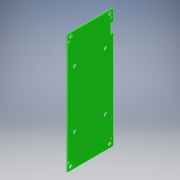
# Autodesk Inventor part: SP01
Saved by Autodesk Inventor 2022 (Build 260153000, 153)
## iProperties
Created: 2021-09-09
Part Number: SP01
Material: Acetal Resin, Black
Document SubType Name: Modeling
Designer: Bowen O'Steen
Density: 1.425 g/cm^3
Appearance: Dark Green
Author: Bowen O'Steen
Autodesk Inventor part; units mm, degrees
ref_plane "YZ Plane" through (0, 0, 0) normal (1, 0, 0) x (0, 1, 0)
ref_plane "XZ Plane" through (0, 0, 0) normal (0, 1, 0) x (-1, 0, 0)
ref_plane "XY Plane" through (0, 0, 0) normal (0, 0, 1) x (1, 0, 0)
sketch "Sketch1" plane through (0, 0, 0) normal (1, 0, 0) x (0, 1, 0)
  line L0 (50, 41.5) -> (-50, 41.5)
  line L1 (-50, 41.5) -> (-50, -41.5)
  line L2 (-50, -41.5) -> (50, -41.5)
  line L3 (50, -41.5) -> (50, 41.5)
  point P0 (0, 0)
  point P1 (50, 0)
  point P2 (0, -41.5)
  dimension "d0" = 100
  dimension "d1" = 83
  constraints: 8 end point, 2 midpoint, 2 parallel, 1 horizontal, 1 horizontal alignment, 1 perpendicular, 1 vertical alignment
  measures "d0" distance of L1.end L2.end
  measures "d1" distance of L2.end L0.start
extrude "Extrusion1" add sketch "Sketch1" along normal blind 1.6
sketch "Sketch12" plane through (0, 50, 41.5) normal (0, 1, 0) x (1, 0, 0)
  line L0 (0, 83) -> (0, 0) projected
  line L1 (0, 0) -> (1.6, 0) projected
  line L2 (1.6, 83) -> (1.6, 0) projected
  line L3 (0, 83) -> (1.6, 83) projected
  point P0 (0, 41.5)
extrude "Extrusion3" add sketch "Sketch12" along normal blind 56.75
sketch "Sketch13" plane through (0, -50, -41.5) normal (0, -1, 0) x (1, 0, 0)
  line L0 (0, 83) -> (0, 0) projected
  line L1 (0, 0) -> (1.6, 0) projected
  line L2 (1.6, 83) -> (1.6, 0) projected
  line L3 (0, 83) -> (1.6, 83) projected
  point P0 (0, 41.5)
extrude "Extrusion4" add sketch "Sketch13" along normal blind 56.75
sketch "Sketch16" plane through (0, 0, 0) normal (-1, 0, 0) x (0, 0, 1)
  line L0 (41.5, -106.75) -> (41.5, 106.75) projected
  line L1 (-41.5, 106.75) -> (41.5, 106.75) projected
  line L2 (-41.5, 106.75) -> (-41.5, -106.75) projected
  line L3 (41.5, -106.75) -> (-41.5, -106.75) projected
  line L4 (0, 0) -> (-25, 0) construction
  point P0 (35, -100.75)
  point P1 (-35, -100.75)
  point P2 (35, 100.75)
  point P3 (-35, 100.75)
  dimension "d168" = 70
  dimension "d169" = 6
  dimension "d170" = 35
  constraints: 2 end point, 2 symmetric about line, 1 horizontal, 1 horizontal alignment
  measures "d168" distance of point (-35, -100.75) point (35, -100.75)
  measures "d169" distance from line of L3 point (35, -100.75)
  measures "d170" horizontal distance of L4.start point (-35, -100.75)
hole "Hole8" at (0, -100.75, 35) at (0, -100.75, -35) at (0, 100.75, 35) at (0, 100.75, -35) direction (1, 0, 0) diameter 6 end through all
sketch "Sketch19" plane through (0, 0, 0) normal (-1, 0, 0) x (0, 0, 1)
  circle A0 centre (-27.5, 51.25) radius 3 construction
  line L0 (-39, 76.75) -> (-39, 72) construction
  line L1 (-39, 76.75) -> (-39, 81.5) construction
  line L2 (-41.5, 106.75) -> (-41.5, -106.75) construction
  line L3 (-41.5, 106.75) -> (41.5, 106.75) projected
  point P0 (0, 0)
  dimension "d194" = 4.75
  dimension "d195" = 4.75
  dimension "d203" = 25.25
  dimension "d204" = 2.5
  constraints: 4 end point, 2 coincident, 1 parallel, 1 vertical alignment
  measures "d194" distance of L0.start L0.end
  measures "d195" distance of L0.start L1.end
  measures "d203" distance from line of L3 point (-39, 81.5)
  measures "d204" distance from line of L2 point (-39, 81.5)
hole "Hole9" at (0, 72, -39) at (0, 81.5, -39) direction (1, 0, 0) diameter 2.6 end through all clearance for "Flat Head Machine Screw" size "M2" standard "Ansi Metric M Profile"
sketch "Sketch21" plane through (0, 0, 0) normal (-1, 0, 0) x (0, 0, 1)
  line L0 (-41.5, 106.75) -> (-41.5, -106.75) projected
  line L1 (-41.5, 85.75) -> (-36.5, 85.75)
  line L2 (-36.5, 85.75) -> (-36.5, 67.75)
  line L3 (-36.5, 67.75) -> (-41.5, 67.75)
  line L4 (-41.5, 67.75) -> (-41.5, 85.75)
  line L5 (-41.5, 106.75) -> (41.5, 106.75) projected
  point P0 (0, 0)
  point P1 (-41.5, 67.75)
  dimension "d205" = 5
  dimension "d206" = 21
  dimension "d207" = 18
  constraints: 8 end point, 2 parallel, 1 horizontal, 1 perpendicular, 1 point on line
  measures "d205" distance of L2.end L3.end
  measures "d206" distance between parallel lines of L5 L1
  measures "d207" distance of L1.end L2.end
extrude "Extrusion5" cut sketch "Sketch21" against normal through all
sketch "Sketch23" plane through (0, 0, 0) normal (-1, 0, 0) x (0, 0, 1)
  circle A0 centre (-35, 100.75) radius 3 projected
  line L0 (0, 0) -> (-12.2775, 0) construction
  point P0 (38, 93.75)
  point P1 (-38, 93.75)
  point P2 (38, -93.75)
  point P3 (-38, -93.75)
  dimension "d220" = 76
  dimension "d221" = 38
  dimension "d229" = 7
  constraints: 2 end point, 2 symmetric about line, 1 horizontal, 1 horizontal alignment
  measures "d220" distance of point (-38, 93.75) point (38, 93.75)
  measures "d221" horizontal distance of L0.start point (-38, 93.75)
  measures "d229" vertical distance of point (-38, 93.75) A0.centre
hole "Hole11" at (0, 93.75, 38) at (0, 93.75, -38) at (0, -93.75, 38) at (0, -93.75, -38) direction (1, 0, 0) diameter 3.454 end through all clearance for "Flat Head Machine Screw (82)" size "#4" standard "Ansi Unified Screw Threads"
sketch "Sketch24" plane through (1.6, 0, 0) normal (1, 0, 0) x (0, 0, -1)
  circle A0 centre (-38, -93.75) radius 1.727 projected
  circle A1 centre (-38, 93.75) radius 1.727 projected
  circle A2 centre (38, 93.75) radius 1.727 projected
  circle A3 centre (38, -93.75) radius 1.727 projected
  line L0 (41.5, 67.75) -> (36.5, 67.75) projected
  line L1 (36.5, 67.75) -> (36.5, 85.75) projected
  line L2 (36.5, 85.75) -> (41.5, 85.75) projected
  line L3 (41.5, 106.75) -> (41.5, 85.75) projected
  line L4 (-41.5, 106.75) -> (41.5, 106.75) projected
  line L5 (-41.5, -106.75) -> (-41.5, 106.75) projected
  line L6 (41.5, -106.75) -> (-41.5, -106.75) projected
  line L7 (41.5, 67.75) -> (41.5, -106.75) projected
  circle A4 centre (35, 100.75) radius 3 projected
  circle A5 centre (35, -100.75) radius 3 projected
  circle A6 centre (-35, -100.75) radius 3 projected
  circle A7 centre (-35, 100.75) radius 3 projected
  line L8 (-41.5, 106.75) -> (-41.5, 93)
  line L9 (-41.5, -106.75) -> (-41.5, 106.75) projected
  line L10 (-41.5, 93) -> (-41.5, 53.25)
  line L11 (-41.5, 53.25) -> (-41.5, 45)
  line L12 (-41.5, 45) -> (-41.5, 5.25)
  line L13 (-41.5, 5.25) -> (-41.5, -8.25)
  line L14 (-41.5, -8.25) -> (41.5, -8.25)
  line L15 (41.5, 67.75) -> (41.5, -106.75) projected
  line L16 (-41.5, -106.75) -> (-41.5, -93)
  line L17 (-41.5, -93) -> (-41.5, -53.25)
  line L18 (-41.5, -53.25) -> (41.5, -53.25)
  line L19 (-41.5, -93) -> (41.5, -93)
  line L20 (-41.5, 5.25) -> (41.5, 5.25)
  line L21 (-41.5, 45) -> (41.5, 45)
  line L22 (-41.5, 53.25) -> (41.5, 53.25)
  line L23 (-41.5, 93) -> (41.5, 93)
  line L24 (41.5, 106.75) -> (41.5, 85.75) projected
  line L25 (-41.5, -53.25) -> (-41.5, -45)
  line L26 (-41.5, -45) -> (41.5, -45)
  line L27 (-41.5, 5.25) -> (-41.5, 4.75)
  line L28 (-41.5, 4.75) -> (41.5, 4.75)
  line L29 (-41.5, -8.25) -> (-41.5, -7.75)
  line L30 (-41.5, -7.75) -> (41.5, -7.75)
  line L31 (0, 106.75) -> (0, -106.75)
  line L32 (-41.5, -106.75) -> (41.5, -106.75) projected
  line L33 (-34.55, 53.275) -> (34.55, 53.275)
  line L34 (34.55, 53.275) -> (34.55, 92.975)
  line L35 (34.55, 92.975) -> (-34.55, 92.975)
  line L36 (-34.55, 92.975) -> (-34.55, 53.275)
  line L37 (-34.55, 53.275) -> (34.55, 92.975) construction
  line L38 (34.55, 53.275) -> (-34.55, 92.975) construction
  line L39 (-34.55, 5.275) -> (34.55, 5.275)
  line L40 (34.55, 5.275) -> (34.55, 44.975)
  line L41 (34.55, 44.975) -> (-34.55, 44.975)
  line L42 (-34.55, 44.975) -> (-34.55, 5.275)
  line L43 (-34.55, 5.275) -> (34.55, 44.975) construction
  line L44 (34.55, 5.275) -> (-34.55, 44.975) construction
  line L45 (-34.55, -94.475) -> (34.55, -94.475)
  line L46 (34.55, -94.475) -> (34.55, -54.775)
  line L47 (34.55, -54.775) -> (-34.55, -54.775)
  line L48 (-34.55, -54.775) -> (-34.55, -94.475)
  line L49 (-34.55, -94.475) -> (34.55, -54.775) construction
  line L50 (34.55, -94.475) -> (-34.55, -54.775) construction
  line L51 (0, -45) -> (0, -25.25)
  line L52 (-34.55, -45.1) -> (34.55, -45.1)
  line L53 (34.55, -45.1) -> (34.55, -5.4)
  line L54 (34.55, -5.4) -> (-34.55, -5.4)
  line L55 (-34.55, -5.4) -> (-34.55, -45.1)
  line L56 (-34.55, -45.1) -> (34.55, -5.4) construction
  line L57 (34.55, -45.1) -> (-34.55, -5.4) construction
  line L58 (41.5, 106.75) -> (-41.5, 106.75) projected
  line L59 (-41.5, 106.75) -> (-34.55, 106.75)
  line L60 (-41.5, 4.75) -> (-32.5, 4.75)
  line L61 (-32.5, 4.75) -> (-32.5, -7.75)
  line L62 (32.5, 4.75) -> (32.5, -7.75)
  point P0 (0, 0)
  point P1 (0, 73.125)
  point P2 (0, 25.125)
  point P3 (0, -74.625)
  point P4 (32.5, -7.75)
  dimension "d230" = 13.75
  dimension "d231" = 39.75
  dimension "d232" = 8.25
  dimension "d233" = 39.75
  dimension "d234" = 13.5
  dimension "d235" = 13.75
  dimension "d236" = 39.75
  dimension "d238" = 8.25
  dimension "d239" = 0.5
  dimension "d240" = 0.5
  dimension "d241" = 69.1
  dimension "d242" = 39.7
  dimension "d243" = 39.7
  dimension "d244" = 39.7
  dimension "d245" = 36.75
  dimension "d246" = 19.75
  dimension "d247" = 69.1
  dimension "d248" = 39.7
  dimension "d249" = 69.1
  dimension "d250" = 9
  constraints: 100 end point, 30 point on line, 14 perpendicular, 11 midpoint, 9 parallel, 4 horizontal, 2 symmetric about line
  measures "d230" distance of L4.start L8.end
  measures "d231" distance of L8.end L10.end
  measures "d232" distance of L10.end L11.end
  measures "d233" distance of L11.end L12.end
  measures "d234" distance of L12.end L13.end
  measures "d235" distance of L5.start L16.end
  measures "d236" distance of L16.end L17.end
  measures "d238" distance of L17.end L25.end
  measures "d239" distance of L12.end L27.end
  measures "d240" distance of L13.end L29.end
  measures "d241" distance of L35.end L34.end
  measures "d242" distance of L34.end L33.end
  measures "d243" distance of L40.end L39.end
  measures "d244" distance of L46.end L45.end
  measures "d245" distance between parallel lines of L26 L14
  measures "d246" distance of L51.start L51.end
  measures "d247" distance of L54.end L53.end
  measures "d248" distance of L53.end L52.end
  measures "d249" distance of L33.start L33.end
  measures "d250" distance of L27.end L60.end
extrude "Extrusion6" cut sketch "Sketch24" against normal blind 10 contours L28 L31 L54 L61 | L61 L54 L31 L30 | L31 L54 L62 L30 | L28 L62 L54 L31
extrude "Extrusion7" add sketch "Sketch24" against normal blind 1.6 contours L28 L31 L54 L61 | L61 L54 L31 L30 | L31 L54 L62 L30 | L28 L62 L54 L31
sketch "Sketch25" plane through (0, 0, 0) normal (-1, 0, 0) x (0, 0, 1)
  line L0 (41.5, -106.75) -> (-41.5, -106.75) projected
  line L1 (41.5, -106.75) -> (41.5, 106.75) projected
  line L2 (0, -106.75) -> (0, -100.8684)
  line L3 (-41.5, 106.75) -> (41.5, 106.75) projected
  line L4 (50, -53.6437) -> (50.1814, -53.6437)
  line L5 (50, -54.25) -> (51.6, -54.25)
  point P0 (0, 0)
  point P1 (27.5, -50.95)
  point P2 (-27.5, -50.95)
  point P3 (27.5, 51.2)
  point P4 (-27.5, 51.2)
  dimension "d255" = 55.8
  dimension "d256" = 14
  dimension "d257" = 55.55
  dimension "d265" = 14
  constraints: 6 end point, 2 horizontal, 2 symmetric about line, 1 midpoint, 1 vertical, 4 other
  measures "d255" distance from line of L0 point (27.5, -50.95)
  measures "d256" distance from line of L1 point (27.5, -50.95)
  measures "d257" distance from line of L3 point (27.5, 51.2)
  measures "d265" distance from line of L1 point (27.5, 51.2)
hole "Hole12" at (0, -50.95, 27.5) at (0, -50.95, -27.5) at (0, 51.2, 27.5) at (0, 51.2, -27.5) direction (1, 0, 0) diameter 6 end through all
sketch "Sketch26" plane through (0, 0, 0) normal (-1, 0, 0) x (0, 0, 1)
  line L0 (0, 0) -> (0, 213.5)
  circle A0 centre (35.5, 0) radius 1.727
  line L1 (32.5, 4.75) -> (32.5, -1.75)
  line L2 (-32.5, -1.75) -> (-32.5, 4.75)
  circle A1 centre (-35.5, 0) radius 1.727
  line L3 (29.5, -4.75) -> (-29.5, -4.75)
  line L4 (-29.5, 7.75) -> (29.5, 7.75)
  line L5 (41.5, -106.75) -> (41.5, 106.75) projected
  line L6 (41.5, -106.75) -> (-41.5, -106.75) projected
  line L7 (-29.5, -4.75) -> (29.5, -4.75)
  line L8 (32.5, -1.75) -> (32.5, 4.75)
  line L9 (29.5, 7.75) -> (-29.5, 7.75)
  line L10 (-32.5, 4.75) -> (-32.5, -1.75)
  arc A2 (-29.5, 7.75) -> (-32.5, 4.75) centre (-29.5, 4.75) ccw
  arc A3 (-32.5, -1.75) -> (-29.5, -4.75) centre (-29.5, -1.75) ccw
  arc A4 (29.5, -4.75) -> (32.5, -1.75) centre (29.5, -1.75) ccw
  arc A5 (32.5, 4.75) -> (29.5, 7.75) centre (29.5, 4.75) ccw
  point P0 (32.5, 7.75)
  point P1 (32.5, -4.75)
  point P2 (-32.5, 7.75)
  dimension "d266" = 65
  dimension "d267" = 12.5
  dimension "d268" = 3
  constraints: 18 end point, 8 point on circle, 8 tangent, 6 centre point, 6 point on line, 3 equal radius, 2 parallel, 1 horizontal, 1 perpendicular
  measures "d266" distance of point (-32.5, 7.75) point (32.5, 7.75)
  measures "d267" distance of point (32.5, 7.75) point (32.5, -4.75)
  measures "d268" radius of A2
equation "\"d170\" = 0.5 * d168"
equation "\"d195\" = d194"
equation "\"d221\" = 0.5 * d220"
body "Solid1"
